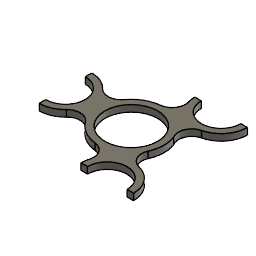
29p3 (Autodesk Fusion 360 design; units mm, degrees)
part number: 2026-08-29-11-21-32-377
Autodesk Fusion 360 part; units mm, degrees
sketch "Sketch1" plane through (0, 0, 0) normal (0, 1, 0) x (1, 0, 0)
  circle A0 centre (0, 0) radius 40
  arc A1 (59.1838, 47.6685) -> (46.7732, 17.6712) centre (63.7757, 28.2028) ccw
  arc A2 (-71, 27.55) -> (-40.3571, 29.5178) centre (-56.5, 41.3249) ccw
  arc A3 (-5.3851, 49.7092) -> (11.6406, 75.2619) centre (-7.5392, 69.5928) ccw
  arc A4 (-40.3571, -29.5178) -> (-71, -27.55) centre (-56.5, -41.3249) ccw
  arc A5 (11.6406, -75.2619) -> (-5.3851, -49.7092) centre (-7.5392, -69.5928) ccw
  arc A6 (45.7425, -20.1898) -> (59.3596, -47.7104) centre (64.0395, -28.2657) ccw
  arc A7 (-40.3571, -29.5178) -> (-5.3851, -49.7092) centre (0, 0) ccw
  arc A8 (45.7425, -20.1898) -> (44.5444, 22.7111) centre (0, 0) ccw
  arc A9 (-5.3851, 49.7092) -> (-40.3571, 29.5178) centre (0, 0) ccw
  arc A10 (-71, 27.55) -> (-100, 40) centre (-100, 0) ccw
  arc A11 (-100, -40) -> (-71, -27.55) centre (-100, 0) ccw
  arc A12 (-100, -30) -> (-100, 30) centre (-100, 0) ccw
  arc A13 (11.6406, -75.2619) -> (10, -86.6) centre (50, -86.6) ccw
  arc A14 (90, -86.6) -> (59.3596, -47.7104) centre (50, -86.6) ccw
  arc A15 (80, -86.6) -> (20, -86.6) centre (50, -86.6) ccw
  arc A16 (59.1838, 47.6685) -> (90, 86.6) centre (50, 86.6) ccw
  arc A17 (10, 86.6) -> (11.6406, 75.2619) centre (50, 86.6) ccw
  arc A18 (20, 86.6) -> (80, 86.6) centre (50, 86.6) ccw
  line L0 (10, 86.6) -> (90, 86.6)
  line L1 (-100, 40) -> (-100, -40)
  line L2 (10, -86.6) -> (90, -86.6)
  point P0 (50, 86.6)
  point P1 (50, -86.6)
  point P2 (50, 86.6)
  dimension "d1" = 80
  dimension "d2" = 100
  dimension "d3" = 60
  dimension "d4" = 80
  dimension "d5" = 60
  dimension "d6" = 80
  dimension "d9" = 50
  dimension "d10" = 86.6
  dimension "d13" = 60
  dimension "d14" = 80
  dimension "d15" = 100
  dimension "d16" = 50
  dimension "d17" = 86.6
  dimension "d18" = 20
  constraint coincident A0.centre A7.centre
  constraint concentric A13 A15
  constraint concentric A16 A18
  constraint concentric A10 A12
  constraint coincident A1.end A8
  constraint tangent A2 A9
  constraint tangent A3 A9
  constraint tangent A4 A7
  constraint tangent A5 A7
  constraint tangent A6 A14
  constraint tangent A1 A16
  constraint equal A1 A6
  constraint equal A5 A6
  constraint equal A4 A5
  constraint equal A2 A4
  constraint equal A1 A3
  constraint tangent A3 A17
  constraint tangent A2 A10
  constraint tangent A4 A11
  constraint tangent A5 A13
  constraint tangent A6 A8
  constraint concentric A7 A9
  constraint coincident A1 A8.end
  constraint concentric A8 A9
  constraint concentric A10 A11
  constraint coincident P2 P0
  constraint coincident P1 A13.centre
  constraint concentric A13 A14
  constraint concentric A16 A17
  constraint horizontal L0
  constraint perpendicular L0 L1
  constraint perpendicular L1 L2
  constraint coincident L0 P2
  measures "d1" diameter of A0
  measures "d2" diameter of A8
  measures "d3" diameter of A15
  measures "d4" diameter of A13
  measures "d5" diameter of A18
  measures "d6" diameter of A16
  measures "d9" horizontal distance of A0.centre P0
  measures "d10" vertical distance of A0.centre P0
  measures "d13" diameter of A12
  measures "d14" diameter of A10
  measures "d15" distance of A0.centre A10.centre
  measures "d16" horizontal distance of A0.centre P1
  measures "d17" vertical distance of A0.centre P1
  measures "d18" radius of A1
extrude "Extrude1" add sketch "Sketch1" along normal blind 10 contours A1 A2 A3 A4 A5 A6 A7 A8 A9 A10 A11 A12 A13 A14 A15 A16 A17 A18 L0 L1 L2
